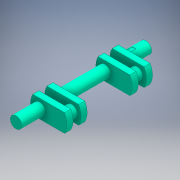
# Autodesk Inventor part: Albero a gomito
Saved by Autodesk Inventor 2016 (Build 200138000, 138)
## iProperties
Created: 2016-09-11
Part Number: Albero a gomito
Material: Generic
Document SubType Name: Modeling
Designer: Muhammad
Density: 1 g/cm^3
Appearance: Default
Author: Muhammad
Autodesk Inventor part; units mm, degrees
ref_plane "YZ Plane" through (0, 0, 0) normal (1, 0, 0) x (0, 1, 0)
sketch "Sketch1" plane through (0, 0, 0) normal (0, 1, 0) x (-1, 0, 0)
  circle A0 centre (0, 0) radius 6
  dimension "d10" = 12
  constraints: 1 centre point, 1 coincident
  measures "d10" diameter of A0
extrude "Extrusion1" add sketch "Sketch1" along normal blind 24.64
sketch "Sketch2" plane through (0, 24.64, 0) normal (0, 1, 0) x (1, 0, 0)
  line L0 (0, 0) -> (9.4, 0) construction
  line L1 (9.4, 0) -> (9.4, -9.4) construction
  line L2 (9.4, -9.4) -> (9.4, 9.4) construction
  line L3 (9.4, 9.4) -> (-7.1118, 9.4) construction
  line L4 (-7.1118, -9.4) -> (25.9118, -9.4)
  line L5 (-7.1118, 9.4) -> (25.9118, 9.4)
  arc A0 (-7.1118, 9.4) -> (-7.1118, -9.4) centre (9.4, 0) ccw
  arc A1 (25.9118, -9.4) -> (25.9118, 9.4) centre (9.4, 0) ccw
  dimension "d3" = 9.4
  dimension "d5" = 9.4
  dimension "d6" = 18.8
  constraints: 12 end point, 4 point on circle, 2 centre point, 2 horizontal, 1 coincident, 1 parallel, 1 perpendicular, 1 point on line, 1 vertical
  measures "d3" distance of L0.start L0.end
  measures "d5" distance of L1.start L1.end
  measures "d6" distance of L1.end L2.end
extrude "Extrusion2" add sketch "Sketch2" along normal blind 6.35
sketch "Sketch3" plane through (0, 30.99, 0) normal (0, 1, 0) x (1, 0, 0)
  arc A0 (25.9118, -9.4) -> (25.9118, 9.4) centre (9.4, 0) ccw construction
  line L0 (28.4, 0) -> (-9.6, 0) construction
  arc A1 (-7.1118, 9.4) -> (-7.1118, -9.4) centre (9.4, 0) ccw construction
  line L1 (9.4, 0) -> (18.8, 0) construction
  circle A2 centre (18.8, 0) radius 6
  point P0 (0, 0)
  dimension "d9" = 9.4
  dimension "d11" = 12
  constraints: 4 end point, 2 point on circle, 1 centre point, 1 coincident, 1 horizontal, 1 point on line
  measures "d9" distance of L1.start L1.end
  measures "d11" diameter of A2
extrude "Extrusion3" add sketch "Sketch3" along normal blind 8.3
sketch "Sketch4" plane through (18.8, 39.29, 0) normal (0, 1, 0) x (1, 0, 0)
  line L0 (-18.8, 0) -> (-9.4, 0) construction
  line L1 (-25.9118, -9.4) -> (7.1118, -9.4) projected
  arc A0 (7.1118, -9.4) -> (7.1118, 9.4) centre (-9.4, 0) ccw projected
  line L2 (-25.9118, -9.4) -> (7.1118, -9.4)
  arc A1 (-25.9118, 9.4) -> (-25.9118, -9.4) centre (-9.4, 0) ccw projected
  line L3 (-25.9118, 9.4) -> (7.1118, 9.4)
  arc A2 (-25.9118, 9.4) -> (-25.9118, -9.4) centre (-8.6906, 0) ccw
  arc A3 (7.1118, -9.4) -> (7.1118, 9.4) centre (-9.4, 0) ccw
  constraints: 6 end point, 4 point on circle, 2 centre point, 2 horizontal, 1 collinear
extrude "Extrusion4" add sketch "Sketch4" along normal blind 6.35
sketch "Sketch5" plane through (18.8, 45.64, 0) normal (0, 1, 0) x (1, 0, 0)
  circle A0 centre (-18.8, 0) radius 6
  constraints: 1 centre point, 1 coincident
extrude "Extrusion5" add sketch "Sketch5" along normal blind 47
ref_plane "Work Plane1" through (0, 69.14, 0) normal (0, 1, 0) x (-1, 0, 0)
mirror "Mirror1" about plane through (0, 69.14, 0) normal (0, 1, 0) of "Extrusion4", "Extrusion3", "Extrusion2"
sketch "Sketch6" plane through (-7.1118, 113.64, -9.4) normal (0, 1, 0) x (1, 0, 0)
  circle A0 centre (7.1118, -9.4) radius 6
  constraints: 1 centre point, 1 coincident
extrude "Extrusion6" add sketch "Sketch6" along normal blind 21.59
sketch "Sketch7" plane through (0, 0, 0) normal (0, 0, 1) x (1, 0, 0)
  line L0 (-6, 0) -> (6, 0) construction
  line L1 (-6, 0) -> (-6, 3.1) construction
  line L2 (-6, 0) -> (-6, 24.64) construction
  line L3 (-6, 3.1) -> (-6, 13.9633) construction
  line L4 (-6, 6.3213) -> (-6.1058, 6.6118) construction
  line L5 (-6, 6.3213) -> (-6, 12.9578) construction
  line L6 (-4, 3.1) -> (-6.1349, 7.8288)
  line L7 (-4, 3.1) -> (-2, 3.1) construction
  line L8 (-4, 3.1) -> (-6, 2.1971)
  line L9 (-6, 2.1971) -> (-6.1349, 7.8288)
  point P0 (0, 0)
  constraints: 16 end point, 6 point on line, 1 horizontal
extrude "Extrusion7" cut sketch "Sketch7" along normal through all both and the other way through all
ref_plane "Work Plane2" through (0, 0, 6) normal (0, 0, 1) x (1, 0, 0)
sketch "Sketch8" plane through (0, 0, 6) normal (0, 0, 1) x (1, 0, 0)
  line L0 (6, 135.23) -> (-6, 135.23) construction
  line L1 (0, 135.23) -> (0, 122.73) construction
  line L2 (0, 122.73) -> (0, 119.73) construction
  line L3 (2, 116.73) -> (-2, 116.73)
  line L4 (-2, 116.73) -> (-2, 122.73)
  line L5 (-2, 122.73) -> (2, 122.73)
  line L6 (2, 122.73) -> (2, 116.73)
  line L7 (2, 116.73) -> (-2, 122.73) construction
  line L8 (-2, 116.73) -> (2, 122.73) construction
  point P0 (0, 0)
  dimension "d29" = 12.5
  dimension "d30" = 3
  dimension "d31" = 4
  constraints: 16 end point, 3 midpoint, 2 parallel, 2 vertical, 1 horizontal, 1 perpendicular
  measures "d29" distance of L1.start L1.end
  measures "d30" distance of L1.end L2.end
  measures "d31" distance of L4.end L5.end
extrude "Extrusion8" cut sketch "Sketch8" against normal blind 0.5
body "Solid1"
